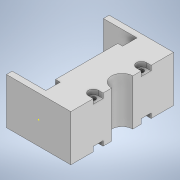
# Autodesk Inventor part: Relaxation chamber holder
Saved by Autodesk Inventor 2022 (Build 260153000, 153)
## iProperties
Created: 2021-11-09
Part Number: Relaxation chamber holder
Material: Generic
Document SubType Name: Modeling
Designer: Emazuddin Alif
Density: 1 g/cm^3
Appearance: Default
Author: Emazuddin Alif
Autodesk Inventor part; units mm, degrees
ref_plane "YZ Plane" through (0, 0, 0) normal (1, 0, 0) x (0, 1, 0)
ref_plane "XZ Plane" through (0, 0, 0) normal (0, 1, 0) x (-1, 0, 0)
ref_plane "XY Plane" through (0, 0, 0) normal (0, 0, 1) x (1, 0, 0)
sketch "Sketch1" plane through (0, 0, 0) normal (0, 1, 0) x (-1, 0, 0)
  line L0 (42.545, 67.945) -> (-42.545, 67.945)
  line L1 (-42.545, -67.945) -> (42.545, -67.945)
  line L2 (42.545, 67.945) -> (-42.545, -67.945) construction
  line L3 (-42.545, 67.945) -> (42.545, -67.945) construction
  line L4 (42.545, 60.325) -> (-1.905, 60.325)
  line L5 (-1.905, 60.325) -> (-1.905, 41.275)
  line L6 (36.0369, 0) -> (-87.2324, 0)
  line L7 (42.545, -60.325) -> (-1.905, -60.325)
  line L8 (-1.905, -60.325) -> (-1.905, -41.275)
  line L9 (-1.905, -41.275) -> (4.445, -41.275)
  line L10 (4.445, 41.275) -> (4.445, -41.275)
  line L11 (-1.905, 41.275) -> (4.445, 41.275)
  line L12 (42.545, -67.945) -> (42.545, -60.325)
  line L13 (42.545, 60.325) -> (42.545, 67.945)
  arc A0 (-42.545, -13.97) -> (-42.545, 13.97) centre (-42.545, 0) ccw
  line L14 (-42.545, 67.945) -> (-42.545, 13.97)
  line L15 (-42.545, -13.97) -> (-42.545, -67.945)
  point P0 (0, 0)
  dimension "d0" = 85.09
  dimension "d2" = 7.62
  dimension "d4" = 19.05
  dimension "d5" = 7.62
  dimension "d6" = 6.35
  dimension "d7" = 135.89
  dimension "d8" = 44.45
  dimension "d9" = 27.94
  dimension "d10" = 53.975
  dimension "d11" = 53.975
  constraints: 32 end point, 6 parallel, 4 perpendicular, 3 horizontal, 3 symmetric about line, 2 midpoint, 2 point on circle, 1 centre point, 1 point on line
  measures "d0" distance of L0.start L0.end
  measures "d2" distance between parallel lines of L0 L4
  measures "d4" distance of L4.end L5.end
  measures "d5" distance between parallel lines of L1 L7
  measures "d6" distance between parallel lines of L5 L10
  measures "d7" distance of L0.end L1.start
  measures "d8" distance between parallel lines of L5 L13
  measures "d9" diameter of A0
  measures "d10" distance of L0.end L14.end
  measures "d11" distance of L15.start L1.start
extrude "Extrusion1" add sketch "Sketch1" along normal mid plane 60.96
sketch "Sketch2" plane through (0, 30.48, 0) normal (0, 1, 0) x (1, 0, 0)
  arc A0 (36.195, -25.273) -> (36.195, -38.227) centre (36.195, -31.75) ccw
  line L0 (36.195, -38.227) -> (42.545, -38.227)
  line L1 (36.195, -25.273) -> (42.545, -25.273)
  line L2 (42.545, 13.97) -> (42.545, 67.945) projected
  line L3 (42.545, -38.227) -> (42.545, -25.273)
  line L4 (42.545, -67.945) -> (42.545, -13.97) projected
  line L5 (-51.5832, 0) -> (64.091, 0)
  line L6 (-42.545, -67.945) -> (42.545, -67.945) projected
  arc A1 (36.195, 38.227) -> (36.195, 25.273) centre (36.195, 31.75) ccw
  line L7 (36.195, 38.227) -> (42.545, 38.227)
  line L8 (36.195, 25.273) -> (42.545, 25.273)
  line L9 (42.545, 38.227) -> (42.545, 25.273)
  point P0 (0, 0)
  point P1 (36.195, 47.3075)
  point P2 (36.195, 34.6075)
  point P3 (42.545, 25.273)
  dimension "d15" = 12.954
  dimension "d23" = 67.945
  dimension "d24" = 63.5
  dimension "d25" = 6.35
  dimension "d26" = 12.954
  constraints: 14 end point, 5 symmetric about line, 4 point on circle, 2 centre point, 2 tangent, 1 collinear, 1 horizontal, 1 vertical, 2 other
  measures "d15" diameter of A0
  measures "d23" distance between parallel lines of L6 L5
  measures "d24" diameter of A0.centre L5
  measures "d25" distance of L7.start L7.end
  measures "d26" distance of L7.end L8.end
extrude "Extrusion2" cut sketch "Sketch2" against normal blind 6.35
mirror "Mirror1" about plane through (0, 0, 0) normal (0, 1, 0) of "Extrusion2"
sketch "Sketch3" plane through (0, 24.13, 0) normal (0, 1, 0) x (1, 0, 0)
  arc A0 (36.195, -25.273) -> (36.195, -38.227) centre (36.195, -31.75) ccw projected
  circle A1 centre (36.195, -31.75) radius 3.175
  line L0 (-42.9578, 0) -> (76.8761, 0)
  circle A2 centre (36.195, 31.75) radius 3.175
  point P0 (0, 0)
  dimension "d19" = 6.35
  constraints: 2 centre point, 2 end point, 1 coincident, 1 horizontal, 1 symmetric about line, 1 other
  measures "d19" diameter of A1
extrude "Extrusion3" cut sketch "Sketch3" against normal through all
sketch "Sketch4" plane through (-42.545, 30.48, 67.945) normal (0, 0, 1) x (1, 0, 0)
  point P0 (42.545, -30.48)
body "Solid1"
